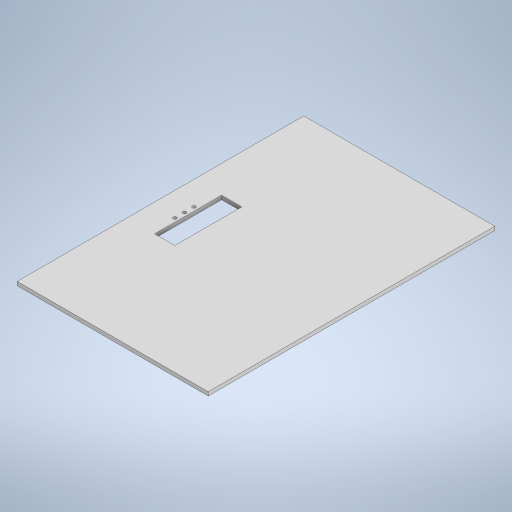
# Autodesk Inventor part: Нижняя полка
Saved by Autodesk Inventor 2023 (Build 270158000, 158)
## iProperties
Created: 2022-05-17
Part Number: Нижняя полка
Material: Типовые
Document SubType Name: Modeling
Designer: avkap
Density: 1 g/cm^3
Appearance: По умолчанию
Author: avkap
Autodesk Inventor part; units mm, degrees
ref_plane "YZ Plane" through (0, 0, 0) normal (1, 0, 0) x (0, 1, 0)
ref_plane "XZ Plane" through (0, 0, 0) normal (0, 1, 0) x (-1, 0, 0)
ref_plane "XY Plane" through (0, 0, 0) normal (0, 0, 1) x (1, 0, 0)
sketch "Эскиз1" plane through (0, 0, 0) normal (0, 1, 0) x (-1, 0, 0)
  line L0 (-200, 0) -> (-600, 0)
  line L1 (-600, 0) -> (-600, -600)
  line L2 (-600, -600) -> (-200, -600)
  line L3 (-200, 0) -> (-250, 0)
  line L4 (-250, 0) -> (-200, 0)
  line L5 (-258, -230) -> (-258, -370)
  line L6 (-300, -230) -> (-258, -230)
  line L7 (-300, -370) -> (-258, -370)
  line L8 (-258, -335) -> (-258, -265)
  line L9 (-300, 0) -> (-200, 0)
  line L10 (-258, -300) -> (-258, -247.9631)
  line L11 (-258, -300) -> (-250, -300)
  line L12 (-250, -300) -> (-250, -280)
  line L13 (-250, -280) -> (-250, -300)
  line L14 (-250, -300) -> (-250, -320)
  circle A0 centre (-250, -320) radius 3.5
  circle A1 centre (-250, -300) radius 3.5
  circle A2 centre (-250, -280) radius 3.5
  line L15 (-300, -300) -> (-300, -230)
  line L16 (-600, 0) -> (-250, 0)
  line L17 (-600, 0) -> (-200, 0)
  line L18 (-200, 0) -> (-200, -600)
  line L19 (-300, -370) -> (-300, -300)
  point P0 (0, 0)
  point P1 (-200, -600)
  point P2 (-200, 0)
  dimension "d1" = 600
  dimension "d16" = 140
  dimension "d17" = 42
  dimension "d23" = 8
  dimension "d24" = 20
  dimension "d26" = 20
  dimension "d27" = 7
  dimension "d28" = 7
  dimension "d29" = 7
  dimension "d30" = 70
  dimension "d31" = 300
  dimension "d33" = 400
  constraints: 40 end point, 5 point on line, 4 perpendicular, 3 centre point, 3 coincident, 3 horizontal, 2 parallel, 1 collinear, 1 midpoint
  measures "d1" distance of L1.end L0.end
  measures "d16" distance of L7.start L6.start
  measures "d17" distance of L6.start L5.start
  measures "d23" distance of L10.start L11.end
  measures "d24" distance of L11.end L12.end
  measures "d26" distance of L11.end L14.end
  measures "d27" diameter of A0
  measures "d28" diameter of A1
  measures "d29" diameter of A2
  measures "d30" distance of L15.start L6.start
  measures "d31" distance of L9.start L15.start
  measures "d33" distance of L0.start L0.end
extrude "Выдавливание2" add sketch "Эскиз1" along normal blind 8
